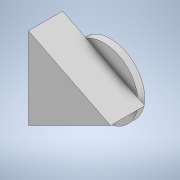
# Autodesk Inventor part: OkBtn
Saved by Autodesk Inventor 2020.1 (Build 241239000, 239)
## iProperties
Created: 2019-09-04
Part Number: OkBtn
Material: Generic
Document SubType Name: Modeling
Designer: matteo.spadetto-1
Density: 1 g/cm^3
Appearance: Default
Author: matteo.spadetto-1
Autodesk Inventor part; units mm, degrees
ref_plane "YZ Plane" through (0, 0, 0) normal (1, 0, 0) x (0, 1, 0)
ref_plane "XZ Plane" through (0, 0, 0) normal (0, 1, 0) x (-1, 0, 0)
ref_plane "XY Plane" through (0, 0, 0) normal (0, 0, 1) x (1, 0, 0)
sketch "Sketch3" plane through (0, 0, 0) normal (0, 0, 1) x (1, 0, 0)
  line L0 (0, 12) -> (0, 0)
  line L1 (0, 0) -> (12, 6)
  line L2 (0, 12) -> (12, 6)
  constraints: 6 end point
extrude "Extrusion4" add sketch "Sketch3" along normal blind 5
sketch "Sketch4" plane through (0, 0, 0) normal (0, 0, -1) x (-1, 0, 0)
  line L0 (0, 0) -> (-12, 6) projected
  circle A0 centre (-6, 6) radius 5
  dimension "d16" = 10
  constraints: 1 centre point
  measures "d16" diameter of A0
extrude "Extrusion5" add sketch "Sketch4" along normal blind 1
body "Solid2"
